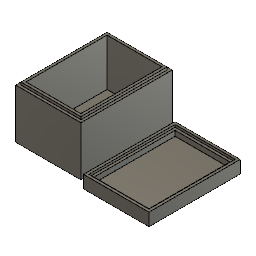
BME590lightbox v3 (Autodesk Fusion 360 design; units mm, degrees)
Autodesk Fusion 360 part; units mm, degrees
sketch "Sketch1" plane through (0, 0, 0) normal (0, 1, 0) x (1, 0, 0)
  line L0 (31.75, 44.45) -> (-31.75, 44.45)
  line L1 (-31.75, 44.45) -> (-31.75, -44.45)
  line L2 (-31.75, -44.45) -> (31.75, -44.45)
  line L3 (31.75, -44.45) -> (31.75, 44.45)
  line L4 (31.75, 44.45) -> (-31.75, -44.45) construction
  line L5 (-31.75, 44.45) -> (31.75, -44.45) construction
  dimension "d1" = 88.9
  dimension "d2" = 63.5
extrude "Extrude1" add sketch "Sketch1" along normal blind 50.8 makes body 1
shell "Shell1" thickness 5.08 removed faces 1 at (-10.5833, 50.8, 14.8167) on bodies 1
sketch "Sketch4" plane through (0, 50.8, 0) normal (0, 1, 0) x (-1, 0, 0)
  line L0 (-26.67, 39.37) -> (26.67, 39.37)
  line L1 (26.67, 39.37) -> (26.67, -39.37)
  line L2 (26.67, -39.37) -> (-26.67, -39.37)
  line L3 (-26.67, -39.37) -> (-26.67, 39.37)
  line L4 (-31.75, 44.45) -> (-31.75, -44.45)
  line L5 (-31.75, -44.45) -> (31.75, -44.45)
  line L6 (31.75, -44.45) -> (31.75, 44.45)
  line L7 (31.75, 44.45) -> (-31.75, 44.45)
  line L8 (29.21, 41.91) -> (-29.21, 41.91)
  line L9 (-29.21, 41.91) -> (-29.21, -41.91)
  line L10 (-29.21, -41.91) -> (29.21, -41.91)
  line L11 (29.21, -41.91) -> (29.21, 41.91)
  dimension "d8" = 2.54
extrude "Extrude2" cut sketch "Sketch4" against normal blind 2.54 contours L4 L5 L6 L7 bodies 1
sketch "Sketch5" plane through (0, 0, 0) normal (0, 1, 0) x (1, 0, 0)
  line L0 (40.64, 38.1) -> (104.14, 38.1)
  line L1 (104.14, 38.1) -> (104.14, -50.8)
  line L2 (104.14, -50.8) -> (40.64, -50.8)
  line L3 (40.64, -50.8) -> (40.64, 38.1)
  dimension "d11" = 63.5
  dimension "d12" = 88.9
extrude "Extrude3" add sketch "Sketch5" along normal blind 10.16 separate body makes body 2
shell "Shell2" thickness 5.08 removed faces 1 at (61.8067, 10.16, -8.4667) on bodies 2
sketch "Sketch6" plane through (0, 10.16, 0) normal (0, 1, 0) x (-1, 0, 0)
  line L0 (-45.72, 45.72) -> (-45.72, -33.02)
  line L1 (-45.72, -33.02) -> (-99.06, -33.02)
  line L2 (-99.06, -33.02) -> (-99.06, 45.72)
  line L3 (-99.06, 45.72) -> (-45.72, 45.72)
  line L4 (-40.64, 50.8) -> (-104.14, 50.8)
  line L5 (-104.14, 50.8) -> (-104.14, -38.1)
  line L6 (-104.14, -38.1) -> (-40.64, -38.1)
  line L7 (-40.64, -38.1) -> (-40.64, 50.8)
  line L8 (-43.18, 48.26) -> (-101.6, 48.26)
  line L9 (-101.6, 48.26) -> (-101.6, -35.56)
  line L10 (-101.6, -35.56) -> (-43.18, -35.56)
  line L11 (-43.18, -35.56) -> (-43.18, 48.26)
  dimension "d16" = 2.54
extrude "Extrude4" add sketch "Sketch6" along normal blind 2.286 contours L4 L5 L6 L7 bodies 2
